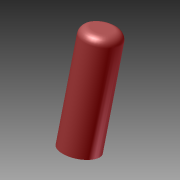
# Autodesk Inventor part: GC-actuator
Saved by Autodesk Inventor 2011 SP1 (Build 150282100, 282)
## iProperties
Created: 2013-12-24
Part Number: GC-actuator
Catalog Web Link: www.cadenas.de
Description: G Series - Ultra-Miniature Fully Illuminated Toggles - actuator-
Vendor: NKKSWITCHES
Document SubType Name: Modeling
Designer: PARTuser1
Manufacturer: NKKSWITCHES
Density: 1 g/cm^3
Category: PARTsolutions
Company: NKKSWITCHES
Title: GC-actuator
Author: Cadenas PARTsolutions
PSOL_IDENT_0: {$CADENAS_DATA\23d-libs\nkkswitches\toggle\g_ill\parts\g_ill_actuator.prj},224 {VTYP=3D},{NB=GC-actu
PSOL_IDENT_1: ator},{LINA=GC-actuator},{NN=G Series - Ultra-Miniature Fully Illuminated Toggles - actuator},{DATE=
PSOL_IDENT_2: 26.03.2009 08:25:15},{GEOMDATE=26.03.2009 08:25:00},{VERSION=},{LINEID=10},{LINESUBID=-1},{WBVAR=LDS
PSOL_IDENT_3: }  {NB=GC-actuator},{LINA=GC-actuator},{KT=DUMMY},{PN=GC},{SRS=G},{LDS=C},{COLOR=RED},{COLORALG=1.00
PSOL_IDENT_4: ,0.00,0.00,0.00}
CNS_NN: G Series - Ultra-Miniature Fully Illuminated Toggles - actuator
CNS_NB: GC-actuator
CNS_NBSYN: $PN.-actuator
CNS_LINA: GC-actuator
CNS_PN: GC
CNS_SRS: G
CNS_LDS: Red
CNS_COLOR: RED
CNS_COLORALG: 1.00,0.00,0.00,0.00
SUPPLIER: NKKSWITCHES
ARTICLENO: GC-actuator
BOMINFO: GC-actuator
CREATOR: CADENAS GmbH
Autodesk Inventor part; units mm, degrees
sketch "Sketch_1" plane through (0, 0, 0) normal (1, 0, 0) x (0, 1, 0)
  line L0 (0.635, 0) -> (5.293, -1.1614)
  line L1 (5.293, -1.1614) -> (5.1793, -1.6173)
  arc A0 (4.7175, -1.8948) -> (5.1793, -1.6173) centre (4.8096, -1.5251) ccw
  line L2 (4.7175, -1.8948) -> (0.4291, -0.8256)
  line L3 (0.4291, -0.8256) -> (0.635, 0)
  line L4 (0.635, 0) -> (5.293, -1.1614)
  constraints: 10 end point, 2 point on circle, 1 centre point
revolve "Revolution1" add sketch "Sketch_1" angle 360 about axis through (0, 0.635, 0) along (0, -0.9702957, 0.2419219)
ref_plane "to_body_XY" through (0, 0, 0) normal (0, 1, 0) x (1, 0, 0)
ref_plane "to_body_YZ" through (0, 0, 0) normal (1, 0, 0) x (0, 0, -1)
ref_plane "to_body_ZX" through (0, 0, 0) normal (0, 0, -1) x (0, 1, 0)
body "Solid1"
